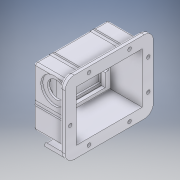
# Autodesk Inventor part: back_board_connector_enclosure
Saved by Autodesk Inventor 2018 (Build 220112000, 112)
## iProperties
Created: 2019-04-16
Part Number: back_board_connector_enclosure
Material: Generic
Document SubType Name: Modeling
Designer: ZEUSLAP
Density: 1 g/cm^3
Appearance: Default
Author: ZEUSLAP
## iProperties of the stored document back_board_connector_enclosure_3DPrint.ipt
Created: 2019-05-12
Part Number: back_board_connector_enclosure_3DPrint
Material: Generic
Document SubType Name: Modeling
Designer: ZEUSLAP
Density: 1 g/cm^3
Appearance: Default
Author: ZEUSLAP
Autodesk Inventor part; units mm, degrees
ref_plane "YZ Plane" through (0, 0, 0) normal (1, 0, 0) x (0, 1, 0)
ref_plane "XZ Plane" through (0, 0, 0) normal (0, 1, 0) x (-1, 0, 0)
sketch "base" plane through (0, 0, 0) normal (0, 0, 1) x (1, 0, 0)
  line L0 (36.5, 29) -> (-36.5, 29)
  line L1 (-36.5, 29) -> (-36.5, -29)
  line L2 (-36.5, -29) -> (36.5, -29)
  line L3 (36.5, -29) -> (36.5, 29)
  line L4 (30, 22) -> (-30, 22)
  line L5 (-30, 22) -> (-30, -21)
  line L6 (-30, -21) -> (30, -21)
  line L7 (30, -21) -> (30, 22)
  line L8 (32.5, -25) -> (-32.5, -25)
  line L9 (-32.5, -25) -> (-32.5, 25)
  line L10 (-32.5, 25) -> (32.5, 25)
  line L11 (32.5, 25) -> (32.5, -25)
  point P0 (0, 0)
  point P1 (-36.5, 0)
  point P2 (0, -29)
  point P3 (0, 22)
  point P4 (0, 29)
  dimension "d56" = 73
  dimension "d57" = 58
  dimension "d58" = 60
  dimension "d59" = 43
  dimension "d60" = 8
  dimension "d75" = 4
  constraints: 24 end point, 6 parallel, 4 midpoint, 3 perpendicular, 2 horizontal, 2 vertical alignment, 1 horizontal alignment, 3 other
  measures "d56" distance of L2.end L1.end
  measures "d57" distance of L1.end L0.end
  measures "d58" distance of L6.end L5.end
  measures "d59" distance of L5.end L4.end
  measures "d60" distance between parallel lines of L2 L6
  measures "d75" distance between parallel lines of L2 L8
extrude "baseExtr" add sketch "base" along normal blind 4 contours L3 L2 L1 L0 | L7 L6 L5 L4 | L8 L9 L10 L11
extrude "shelfExtr" add sketch "base" against normal blind 6 contours L7 L6 L5 L4
extrude "wallsExtr" add sketch "base" against normal blind 29 contours L3 L2 L1 L0
sketch "bluepill" plane through (0, 0, -6) normal (0, 0, -1) x (-1, 0, 0)
  line L0 (-27, -18) -> (27, -18)
  line L1 (27, -18) -> (27, 5)
  line L2 (27, 5) -> (-27, 5)
  line L3 (-27, 5) -> (-27, -18)
  line L4 (-30, -21) -> (30, -21) projected
  line L5 (-25.5, -15.5) -> (18.5, -15.5)
  line L6 (18.5, -15.5) -> (18.5, 2.5)
  line L7 (18.5, 2.5) -> (-25.5, 2.5)
  line L8 (-25.5, 2.5) -> (-25.5, -15.5)
  line L9 (30, 22) -> (-30, 22) projected
  point P0 (0, 0)
  point P1 (-25.5, -6.5)
  point P2 (-27, -6.5)
  point P3 (0, 5)
  point P4 (0, 22)
  dimension "d65" = 54
  dimension "d66" = 23
  dimension "d67" = 3
  dimension "d68" = 44
  dimension "d69" = 18
  dimension "d179" = 1.5
  constraints: 16 end point, 4 midpoint, 4 parallel, 2 horizontal, 2 perpendicular, 1 horizontal alignment, 1 vertical alignment
  measures "d65" distance of L2.end L1.end
  measures "d66" distance of L1.end L0.end
  measures "d67" distance between parallel lines of L0 L4
  measures "d68" distance of L7.end L6.end
  measures "d69" distance of L6.end L5.end
  measures "d179" distance between parallel lines of L8 L3
extrude "boardExtr" cut sketch "bluepill" against normal blind 6
extrude "componentExtr" cut sketch "bluepill" against normal blind 8 contours L8 L7 L6 L5
sketch "Sketch10" plane through (-18.5, 2.5, 0) normal (0, -1, 0) x (1, 0, 0)
  line L0 (0, 0) -> (44, 0) projected
  line L1 (44, 0) -> (44, 2) projected
  line L2 (44, 2) -> (0, 2) projected
  line L3 (0, 0) -> (0, 2) projected
  point P0 (18.5, 0)
extrude "componentSlideExtr" cut sketch "Sketch10" against normal blind 15
sketch "Sketch13" plane through (-27, 5, -6) normal (0, -1, 0) x (1, 0, 0)
  line L0 (54, 6) -> (52.5, 6) construction
  line L1 (54, 6) -> (51, 6)
  line L2 (51, 6) -> (51, 0)
  line L3 (54, 0) -> (0, 0) projected
  line L4 (51, 0) -> (0, 0)
  line L5 (0, 0) -> (0, 6) projected
  line L6 (0, 0) -> (0, 6)
  line L7 (0, 6) -> (51, 6)
  line L8 (54, 6) -> (54, 4)
  line L9 (54, 0) -> (54, 6) projected
  line L10 (54, 4) -> (51, 4)
  point P0 (27, 6)
  dimension "d87" = 3
  dimension "d88" = 90
  dimension "d89" = 2
  constraints: 14 end point, 4 point on line, 3 perpendicular
  measures "d87" distance of L0.start L1.end
  measures "d88" angle of L2 L1
  measures "d89" distance of L0.start L8.end
extrude "boardSlideExtr" cut sketch "Sketch13" against normal blind 13 contours L8 L10 L2 L1 | L2 L3 L5 L7
sketch "Sketch14" plane through (-27, 18, -6) normal (0, -1, 0) x (1, 0, 0)
  line L0 (0, 6) -> (0, 3.5)
  line L1 (0, 6) -> (54, 6) projected
  line L2 (0, 6) -> (54, 6)
  line L3 (54, 6) -> (54, 3.5)
  line L4 (0, 3.5) -> (54, 3.5)
  dimension "d188" = 2.5
  constraints: 8 end point, 2 perpendicular, 1 collinear, 1 parallel, 1 vertical
  measures "d188" distance of L0.start L0.end
extrude "boardBottomSlideExtr" cut sketch "Sketch14" against normal blind 2
sketch "sp16_hole" plane through (-36.5, -29, 4) normal (-1, 0, 0) x (0, 0, 1)
  circle A0 centre (-20, 14.5) radius 13
  line L0 (0, 58) -> (0, 0) projected
  circle A1 centre (-20, 14.5) radius 8.5
  line L1 (-33, 0) -> (0, 0) projected
  point P0 (-4, 29)
  point P1 (0, 29)
  point P2 (-4, 0)
  dimension "d99" = 26
  dimension "d100" = 20
  dimension "d103" = 17
  dimension "d106" = 14.5
  constraints: 2 centre point, 1 coincident, 1 midpoint
  measures "d99" diameter of A0
  measures "d100" distance from line of A0.centre L0
  measures "d103" diameter of A1
  measures "d106" distance from line of L1 A0.centre
extrude "sp16ReceptableExtr" cut sketch "sp16_hole" against normal blind 2 contours A0 | A1
extrude "sp16HoleExtr" cut sketch "sp16_hole" against normal up to surface (4 mm away) contours A1
fillet "enclosure_fillet" radius 2 8 edges at (36.5, -29, -12.5) (0, -29, 4) (-36.5, -29, -12.5) (36.5, 0, 4) (0, 29, 4) (-36.5, 0, 4) (36.5, 29, -12.5) (-36.5, 29, -12.5)
ref_plane "Work Plane1" through (-27, -11, -6) normal (0, 1, 0) x (1, 0, 0)
sketch "Sketch17" plane through (-27, -11, -6) normal (0, 1, 0) x (1, 0, 0)
  line L0 (0, 0) -> (54, 0) projected
  line L1 (0, 0) -> (0, -6) projected
  line L2 (0, -6) -> (54, -6) projected
  line L3 (54, 0) -> (54, -6) projected
  line L4 (0, -6) -> (-1, -6)
  line L5 (-1, -6) -> (-1, 0)
  line L6 (-1, 0) -> (0, 0)
  point P0 (27, -6)
  dimension "d109" = 1
  constraints: 6 end point, 2 perpendicular, 1 horizontal
  measures "d109" distance of L1.end L4.end
extrude "usbSlideExtr" cut sketch "Sketch17" along normal blind 24 contours L1 L4 L5 L6
sketch "lip&screws" plane through (0, 0, -29) normal (0, 0, -1) x (-1, 0, 0)
  line L0 (-32.5, 25) -> (32.5, 25) projected
  line L1 (-32.5, -25) -> (-32.5, 25) projected
  line L2 (32.5, 25) -> (32.5, -25) projected
  line L3 (32.5, -25) -> (-32.5, -25) projected
  line L4 (34.5, 29) -> (-34.5, 29) projected
  arc A0 (-34.5, 29) -> (-36.5, 27) centre (-34.5, 27) ccw projected
  line L5 (-36.5, 27) -> (-36.5, -27) projected
  arc A1 (-36.5, -27) -> (-34.5, -29) centre (-34.5, -27) ccw projected
  line L6 (-34.5, -29) -> (34.5, -29) projected
  arc A2 (34.5, -29) -> (36.5, -27) centre (34.5, -27) ccw projected
  line L7 (36.5, -27) -> (36.5, 27) projected
  arc A3 (36.5, 27) -> (34.5, 29) centre (34.5, 27) ccw projected
  line L8 (-34.5, 36) -> (34.5, 36)
  arc A4 (43.5, 27) -> (34.5, 36) centre (34.5, 27) ccw
  line L9 (43.5, 27) -> (43.5, -27)
  arc A5 (34.5, -36) -> (43.5, -27) centre (34.5, -27) ccw
  line L10 (34.5, -36) -> (-34.5, -36)
  arc A6 (-43.5, -27) -> (-34.5, -36) centre (-34.5, -27) ccw
  line L11 (-43.5, -27) -> (-43.5, 27)
  arc A7 (-34.5, 36) -> (-43.5, 27) centre (-34.5, 27) ccw
  circle A8 centre (20, -31) radius 1.75
  circle A9 centre (-20, -31) radius 1.75
  circle A10 centre (38.5, 5) radius 1.75
  circle A11 centre (20, 31) radius 1.75
  circle A12 centre (-20, 31) radius 1.75
  circle A13 centre (-38.5, 15) radius 1.75
  circle A14 centre (-38.5, -15) radius 1.75
  line L12 (0, -39.6728) -> (0, 44.8826) construction
  line L13 (66.7304, 0) -> (-63.1993, 0) construction
  line L14 (-41.5, -16.7321) -> (-41.5, -13.2679)
  line L15 (-41.5, -13.2679) -> (-38.5, -11.5359)
  line L16 (-38.5, -11.5359) -> (-35.5, -13.2679)
  line L17 (-35.5, -13.2679) -> (-35.5, -16.7321)
  line L18 (-35.5, -16.7321) -> (-38.5, -18.4641)
  line L19 (-38.5, -18.4641) -> (-41.5, -16.7321)
  line L20 (-41.5, 16.7321) -> (-38.5, 18.4641)
  line L21 (-38.5, 18.4641) -> (-35.5, 16.7321)
  line L22 (-35.5, 16.7321) -> (-35.5, 13.2679)
  line L23 (-35.5, 13.2679) -> (-38.5, 11.5359)
  line L24 (-38.5, 11.5359) -> (-41.5, 13.2679)
  line L25 (-41.5, 13.2679) -> (-41.5, 16.7321)
  line L26 (-16.5359, 31) -> (-18.2679, 28)
  line L27 (-18.2679, 28) -> (-21.7321, 28)
  line L28 (-21.7321, 28) -> (-23.4641, 31)
  line L29 (-23.4641, 31) -> (-21.7321, 34)
  line L30 (-21.7321, 34) -> (-18.2679, 34)
  line L31 (-18.2679, 34) -> (-16.5359, 31)
  line L32 (23.4641, 31) -> (21.7321, 28)
  line L33 (21.7321, 28) -> (18.2679, 28)
  line L34 (18.2679, 28) -> (16.5359, 31)
  line L35 (16.5359, 31) -> (18.2679, 34)
  line L36 (18.2679, 34) -> (21.7321, 34)
  line L37 (21.7321, 34) -> (23.4641, 31)
  line L38 (41.5, 6.7321) -> (41.5, 3.2679)
  line L39 (41.5, 3.2679) -> (38.5, 1.5359)
  line L40 (38.5, 1.5359) -> (35.5, 3.2679)
  line L41 (35.5, 3.2679) -> (35.5, 6.7321)
  line L42 (35.5, 6.7321) -> (38.5, 8.4641)
  line L43 (38.5, 8.4641) -> (41.5, 6.7321)
  line L44 (21.7321, -34) -> (18.2679, -34)
  line L45 (18.2679, -34) -> (16.5359, -31)
  line L46 (16.5359, -31) -> (18.2679, -28)
  line L47 (18.2679, -28) -> (21.7321, -28)
  line L48 (21.7321, -28) -> (23.4641, -31)
  line L49 (23.4641, -31) -> (21.7321, -34)
  line L50 (-21.7321, -34) -> (-23.4641, -31)
  line L51 (-23.4641, -31) -> (-21.7321, -28)
  line L52 (-21.7321, -28) -> (-18.2679, -28)
  line L53 (-18.2679, -28) -> (-16.5359, -31)
  line L54 (-16.5359, -31) -> (-18.2679, -34)
  line L55 (-18.2679, -34) -> (-21.7321, -34)
  point P0 (0, 0)
  dimension "d147" = 7
  dimension "d151" = 3.5
  dimension "d152" = 6
  dimension "d153" = 20
  dimension "d154" = 6
  dimension "d155" = 15
  dimension "d158" = 6
  dimension "d159" = 20
  dimension "d160" = 3
  dimension "d161" = 3
  dimension "d162" = 3
  constraints: 96 end point, 11 centre point, 8 point on circle, 7 coincident, 6 equal radius, 5 horizontal, 5 symmetric about line, 3 vertical, 2 collinear, 2 point on line, 100 other
  measures "d147" distance between parallel lines of L8 L4
  measures "d151" diameter of A8
  measures "d152" distance from line of L3 A8.centre
  measures "d153" distance from line of A8.centre L12
  measures "d154" distance from line of L1 A14.centre
  measures "d155" vertical distance of point (0, 0) A13.centre
  measures "d158" distance from line of L2 A10.centre
  measures "d159" distance from line of L0 A10.centre
  measures "d160" distance from line of A14.centre L14
  measures "d161" distance from line of L55 A9.centre
  measures "d162" distance from line of L43 A10.centre
extrude "lipExtr" add sketch "lip&screws" along normal blind 5 contours A3 L7 L42 L41 L40 A2 L6 L48 L47 L46 L53 L52 L51 A1 L5 L18 L17 L16 L23 L22 L21 A0 L4 L28 L27 L26 L34 L33 L32 | L32 L33 L34 L4 | L4 L34 L35 L36 L37 L32 | L42 L43 L38 L39 L40 L7 | L7 L40 L41 L42 | L26 L27 L28 L4 | L4 L28 L29 L30 L31 L26 | L48 L49 L44 L45 L46 L6 | L6 L46 L47 L48 | L21 L22 L23 L5 | L5 L23 L24 L25 L20 L21 | L53 L54 L55 L50 L51 L6 | L6 L51 L52 L53 | L16 L17 L18 L5 | L5 L18 L19 L14 L15 L16 | L8 A4 L9 A5 L10 A6 L11 A7 | A8 | A9 | A10 | A11 | A12 | A13 | A14
fillet "lip_Fillet2" radius 2 17 edges at (0, 36, -29) (-40.864, 33.364, -29) (-43.5, 0, -29) (-40.864, -33.364, -29) (0, -36, -29) (40.864, -33.364, -29) (43.5, 0, -29) (40.864, 33.364, -29) (35.9142, 28.4142, -29) (36.5, 0, -29) (35.9142, -28.4142, -29) (0, -29, -29) (-35.9142, -28.4142, -29) (-36.5, -20.75, -29) (-36.5, 6.25, -29) (-35.9142, 28.4142, -29) (0, 29, -29)
extrude "m3holes" cut sketch "lip&screws" along normal mid plane 10 contours A8 | A9 | A10 | A11 | A12 | A13 | A14
extrude "m3nut_holes" cut sketch "lip&screws" along normal blind 2.5 and the other way blind 50 contours L32 L33 L34 L4 | L4 L34 L35 L36 L37 L32 | L42 L43 L38 L39 L40 L7 | L7 L40 L41 L42 | L26 L27 L28 L4 | L4 L28 L29 L30 L31 L26 | L48 L49 L44 L45 L46 L6 | L6 L46 L47 L48 | L21 L22 L23 L5 | L5 L23 L24 L25 L20 L21 | L53 L54 L55 L50 L51 L6 | L6 L51 L52 L53 | L16 L17 L18 L5 | L5 L18 L19 L14 L15 L16
sketch "Sketch20" plane through (-17.6906, 29, 2) normal (0, 1, 0) x (1, 0, 0)
  line L0 (6.6906, 25.5) -> (28.6906, 25.5)
  line L1 (28.6906, 25.5) -> (28.6906, 3.5)
  line L2 (28.6906, 3.5) -> (6.6906, 3.5)
  line L3 (6.6906, 3.5) -> (6.6906, 25.5)
  line L4 (6.6906, 25.5) -> (28.6906, 3.5) construction
  line L5 (6.6906, 3.5) -> (28.6906, 25.5) construction
  line L6 (-16.8094, 0) -> (-16.8094, 29) construction
  line L7 (0, 29) -> (35.3812, 29) construction
  point P0 (17.6906, 2)
  point P1 (17.6906, 14.5)
  point P2 (17.6906, 14.5)
  point P3 (-16.8094, 14.5)
  point P4 (17.6906, 29)
  dimension "d167" = 22
  dimension "d168" = 22
  constraints: 12 end point, 4 midpoint, 2 parallel, 1 horizontal, 1 horizontal alignment, 1 perpendicular, 1 vertical alignment
  measures "d167" distance of L1.end L2.end
  measures "d168" distance of L0.end L1.end
extrude "stem" add sketch "Sketch20" along normal blind 10
sketch "Sketch21" plane through (-17.6906, 39, 2) normal (0, 1, 0) x (1, 0, 0)
  line L0 (28.6906, 25.5) -> (6.6906, 25.5) projected
  line L1 (6.6906, 25.5) -> (6.6906, 3.5) projected
  line L2 (6.6906, 3.5) -> (28.6906, 3.5) projected
  line L3 (28.6906, 3.5) -> (28.6906, 25.5) projected
  line L4 (28.6906, 25.5) -> (28.6906, 3.5)
  line L5 (28.6906, 3.5) -> (48.6906, 3.5)
  line L6 (48.6906, 3.5) -> (48.6906, 25.5)
  line L7 (48.6906, 25.5) -> (28.6906, 25.5)
  line L8 (6.6906, 3.5) -> (6.6906, 25.5) projected
  line L9 (6.6906, 25.5) -> (6.6906, 3.5)
  line L10 (6.6906, 3.5) -> (-13.3094, 3.5)
  line L11 (-13.3094, 3.5) -> (-13.3094, 25.5)
  line L12 (-13.3094, 25.5) -> (6.6906, 25.5)
  dimension "d180" = 20
  dimension "d181" = 20
  constraints: 16 end point, 5 equal length, 3 perpendicular
  measures "d180" distance of L5.end L2.end
  measures "d181" distance of L1.end L10.end
extrude "tee" add sketch "Sketch21" along normal blind 4
fillet "tee_Fillet5" radius 2 14 edges at (11, 29, -12.5) (0, 29, -1.5) (-11, 29, -12.5) (0, 29, -23.5) (-11, 34, -23.5) (-11, 34, -1.5) (11, 34, -1.5) (11, 34, -23.5) (11, 39, -12.5) (-11, 39, -12.5) (21, 39, -1.5) (-21, 39, -1.5) (21, 39, -23.5) (-21, 39, -23.5)
sketch "Sketch24" plane through (0, 0, -6) normal (0, 0, -1) x (-1, 0, 0)
  line L0 (30, 22) -> (30, -21) projected
  line L1 (30, -21) -> (30, -6)
  line L2 (30, -6) -> (28, -6)
  line L3 (28, 13) -> (28, -11) projected
  line L4 (28, -6) -> (28, -11)
  line L5 (28, -11) -> (27, -11) projected
  line L6 (28, -11) -> (27, -11)
  line L7 (27, -11) -> (27, -18) projected
  line L8 (27, -11) -> (27, -18)
  line L9 (27, -18) -> (20, -18)
  line L10 (27, -18) -> (-27, -18) projected
  line L11 (20, -18) -> (20, -21)
  line L12 (30, -21) -> (-30, -21) projected
  point P0 (0, 0)
  dimension "d189" = 15
  dimension "d190" = 2
  dimension "d191" = 7
  constraints: 14 end point, 4 point on line, 1 collinear, 1 horizontal, 1 perpendicular
  measures "d189" distance of L0.end L1.end
  measures "d190" distance of L1.end L2.end
  measures "d191" distance of L7.end L9.end
extrude "extra_space_for_back_nut" cut sketch "Sketch24" against normal blind 3
fillet "Fillet6" radius 2 4 edges at (-29, -6, -6) (-29, -6, -3) (-20, -19.5, -3) (-20, -19.5, -6)
fillet "Fillet7" radius 1 14 edges at (-19.3518, -21, -5.5811) (-20.7753, -21, -3.4189) (-26, -21, -3) (5.9365, -21, -6) (30, 0.5, -6) (0, 22, -6) (-30, -5.2247, -5.5811) (-30, -6.6482, -3.4189) (-30, -14.4365, -3) (-30, 9, -6) (-30, 0.5, 0) (0, 22, 0) (30, 0.5, 0) (0, -21, 0)
body "Solid3"
